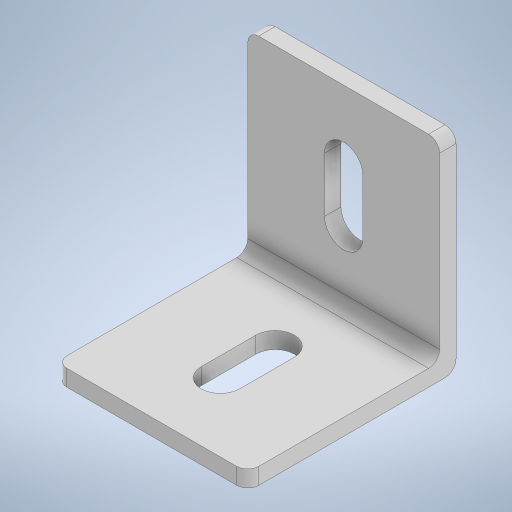
# Autodesk Inventor part: L자 브라켓
Saved by Autodesk Inventor 2023 (Build 270158000, 158)
## iProperties
Created: 2024-02-08
Part Number: L자 브라켓
Material: 일반
Document SubType Name: Modeling
Designer: ps737
Density: 1 g/cm^3
Appearance: 기본값
Author: ps737
Autodesk Inventor part; units mm, degrees
ref_plane "YZ Plane" through (0, 0, 0) normal (1, 0, 0) x (0, 1, 0)
ref_plane "XZ Plane" through (0, 0, 0) normal (0, 1, 0) x (-1, 0, 0)
ref_plane "XY Plane" through (0, 0, 0) normal (0, 0, 1) x (1, 0, 0)
sketch "스케치1" plane through (0, 0, 0) normal (0, 1, 0) x (-1, 0, 0)
  line L0 (8.1082, 12.9394) -> (-22.8918, 12.9394)
  line L1 (-24.8918, 10.9394) -> (-24.8918, -22.0606)
  line L2 (-24.8918, -22.0606) -> (10.1082, -22.0606)
  line L3 (10.1082, -22.0606) -> (10.1082, 10.9394)
  arc A0 (10.1082, 10.9394) -> (8.1082, 12.9394) centre (8.1082, 10.9394) ccw
  arc A1 (-22.8918, 12.9394) -> (-24.8918, 10.9394) centre (-22.8918, 10.9394) ccw
  line L4 (10.1082, -25.0606) -> (-24.8918, -25.0606)
  line L5 (10.1082, -22.0606) -> (10.1082, -25.0606)
  line L6 (-24.8918, -22.0606) -> (-24.8918, -25.0606)
  line L7 (-10.8918, -9.5606) -> (-10.8918, 0.4394)
  line L8 (-3.8918, -9.5606) -> (-3.8918, 0.4394)
  line L9 (-3.8918, 0.4394) -> (-10.8918, 0.4394)
  line L10 (-10.8918, -9.5606) -> (-3.8918, -9.5606)
  arc A2 (-10.8918, -9.5606) -> (-3.8918, -9.5606) centre (-7.3918, -9.5606) ccw
  arc A3 (-3.8918, 0.4394) -> (-10.8918, 0.4394) centre (-7.3918, 0.4394) ccw
  line L11 (-24.8918, 19.0606) -> (-24.8918, -10.9394)
  point P0 (0, 0)
  point P1 (-24.8918, 12.9394)
  point P2 (0, 0)
  point P3 (-3.8918, -4.5606)
  point P4 (-10.8918, -4.5606)
  point P5 (-7.3918, -23.5606)
  point P6 (-7.3918, -22.0606)
  point P7 (-7.3918, -13.0606)
  point P8 (-7.3918, 12.9394)
  point P9 (-7.3918, 3.9394)
  dimension "d0" = 35
  dimension "d1" = 35
  dimension "d2" = 2
  dimension "d3" = 2
  dimension "d14" = 3
  dimension "d20" = 10
  dimension "d21" = 7
  dimension "d22" = 14
  dimension "d23" = 14
  dimension "d24" = 14
  dimension "d26" = 9
  constraints: 24 end point, 10 point on circle, 6 midpoint, 4 centre point, 4 parallel, 4 perpendicular, 4 point on line, 4 tangent, 2 vertical, 1 horizontal
  measures "d0" distance of L2.end L1.end
  measures "d1" distance of L1.end point (-24.892, 12.939)
  measures "d2" radius of A0
  measures "d3" radius of A1
  measures "d14" distance between parallel lines of L4 L2
  measures "d20" distance of L7.start L7.end
  measures "d21" distance of point (-3.892, -4.561) point (-10.892, -4.561)
  measures "d22" distance between parallel lines of L11 L7
  measures "d23" distance from line of point (-7.392, -23.561) L10
  measures "d24" distance between parallel lines of L1 L7
  measures "d26" distance of point (-7.392, 12.939) point (-7.392, 3.939)
extrude "돌출3" add sketch "스케치1" along normal blind 3 contours A0 L3 L2 L1 A1 L0 | L7 L9 L8 L10 | L10 A2 | A3 L9
extrude "돌출4" add sketch "스케치1" along normal blind 38 contours L5 L4 L6 L2
fillet "모깎기2" radius 2 4 edges at (24.8918, 38, -23.5606) (-10.1082, 38, -23.5606) (7.3918, 3, -22.0606) (7.3918, 0, -25.0606)
sketch "스케치6" plane through (24.8918, 2, -25.0606) normal (0, 0, -1) x (-1, 0, 0)
  line L0 (33, 36) -> (2, 36)
  line L1 (0, 34) -> (0, 1)
  line L2 (0, 1) -> (35, 1)
  line L3 (35, 1) -> (35, 34)
  arc A0 (35, 34) -> (33, 36) centre (33, 34) ccw
  arc A1 (2, 36) -> (0, 34) centre (2, 34) ccw
  line L4 (35, -2) -> (0, -2)
  line L5 (35, 1) -> (35, -2)
  line L6 (0, 1) -> (0, -2)
  line L7 (14, 13.5) -> (14, 23.5)
  line L8 (21, 13.5) -> (21, 23.5)
  line L9 (21, 23.5) -> (14, 23.5)
  line L10 (14, 13.5) -> (21, 13.5)
  arc A2 (14, 13.5) -> (21, 13.5) centre (17.5, 13.5) ccw
  arc A3 (21, 23.5) -> (14, 23.5) centre (17.5, 23.5) ccw
  line L11 (0, 42.063) -> (0, 12.063)
  line L12 (0, 0) -> (0, 34) projected
  line L13 (0, -2) -> (35, -2) projected
  point P0 (24.8918, -2)
  point P1 (24.6406, 23.0024)
  point P2 (0, 36)
  point P3 (24.6406, 23.0024)
  point P4 (14, 18.5)
  point P5 (21, 18.5)
  point P6 (17.2488, -0.5)
  point P7 (17.5, 1)
  point P8 (17.5, 10)
  point P9 (17.5, 36)
  point P10 (17.5, 27)
  dimension "d38" = 35
  dimension "d39" = 35
  dimension "d40" = 2
  dimension "d41" = 2
  dimension "d42" = 3
  dimension "d43" = 10
  dimension "d44" = 7
  dimension "d45" = 14
  dimension "d46" = 14
  dimension "d47" = 14
  dimension "d48" = 9
  dimension "d49" = 0
  dimension "d50" = 0
  constraints: 24 end point, 10 point on circle, 6 midpoint, 4 centre point, 4 parallel, 4 perpendicular, 4 point on line, 4 tangent, 2 vertical, 1 horizontal
  measures "d38" distance of L2.end L1.end
  measures "d39" distance of L1.end point (0, 36)
  measures "d40" radius of A0
  measures "d41" radius of A1
  measures "d42" distance between parallel lines of L4 L2
  measures "d43" distance of L7.start L7.end
  measures "d44" distance of point (21, 18.5) point (14, 18.5)
  measures "d45" distance between parallel lines of L11 L7
  measures "d46" distance from line of point (17.249, -0.5) L10
  measures "d47" distance between parallel lines of L1 L7
  measures "d48" distance of point (17.5, 36) point (17.5, 27)
  measures "d49" distance between parallel lines of L12 L1
  measures "d50" distance between parallel lines of L13 L4
extrude "돌출5" cut sketch "스케치6" against normal blind 38 contours L7 L9 L8 L10 | L10 A2 | A3 L9
extrude "돌출6" cut sketch "스케치1" along normal blind 38 contours L7 L9 L8 L10 | L10 A2 | A3 L9
